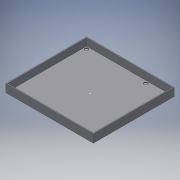
# Autodesk Inventor part: 240621_pt1
Saved by Autodesk Inventor 2016 (Build 200138000, 138)
## iProperties
Created: 2024-06-21
Part Number: 240621_pt1
Material: 일반
Document SubType Name: Modeling
Designer: pc
Density: 1 g/cm^3
Appearance: 기본값
Author: pc
Autodesk Inventor part; units mm, degrees
ref_plane "YZ Plane" through (0, 0, 0) normal (1, 0, 0) x (0, 1, 0)
ref_plane "XZ Plane" through (0, 0, 0) normal (0, 1, 0) x (-1, 0, 0)
ref_plane "XY Plane" through (0, 0, 0) normal (0, 0, 1) x (1, 0, 0)
sketch "스케치1" plane through (0, 0, 0) normal (0, 0, 1) x (1, 0, 0)
  line L0 (65, -60) -> (-65, -60)
  line L1 (-65, -60) -> (-65, 60)
  line L2 (-65, 60) -> (65, 60)
  line L3 (65, 60) -> (65, -60)
  line L4 (65, -60) -> (-65, 60) construction
  line L5 (-65, -60) -> (65, 60) construction
  line L6 (63, 58) -> (-63, 58) construction
  line L7 (-63, 58) -> (-63, -58) construction
  line L8 (-63, -58) -> (63, -58) construction
  line L9 (63, -58) -> (63, 58) construction
  point P0 (0, 0)
  dimension "d0" = 130
  dimension "d1" = 120
  dimension "d2" = 2
  constraints: 20 end point, 4 parallel, 2 midpoint, 2 perpendicular, 1 horizontal, 3 other
  measures "d0" distance of L1.end L2.end
  measures "d1" distance of L0.end L1.end
  measures "d2" distance between parallel lines of L2 L6
extrude "돌출1" add sketch "스케치1" along normal blind 12
shell "쉘1" thickness 1.2 removed faces 1 at (21.6667, 20, 12)
sketch "스케치2" plane through (-63.8, -58.8, 1.2) normal (0, 0, 1) x (1, 0, 0)
  point P0 (63.8, 58.8)
sketch "스케치3" plane through (-63.8, -58.8, 1.2) normal (0, 0, 1) x (1, 0, 0)
  circle A0 centre (92.0039, 113.6118) radius 2.7
  circle A1 centre (4.0037, 3.6486) radius 2.7
  circle A2 centre (4.0037, 113.6118) radius 2.7
  circle A3 centre (124.0062, 3.6486) radius 2.7
  point P0 (63.8, 58.8)
  dimension "d6" = 5.4
  dimension "d7" = 5.4
  dimension "d8" = 5.4
  dimension "d9" = 5.4
  constraints: 4 centre point
  measures "d6" diameter of A0
  measures "d7" diameter of A1
  measures "d8" diameter of A2
  measures "d9" diameter of A3
extrude "돌출2" cut sketch "스케치3" against normal blind 12
